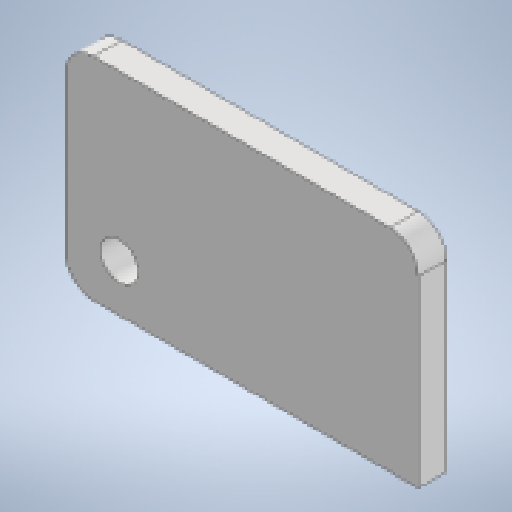
# Autodesk Inventor part: креп_центр_рейки
Saved by Autodesk Inventor 2023.1 (Build 271208000, 208)
## iProperties
Created: 2025-11-24
Part Number: креп_центр_рейки
Material: Типовые
Document SubType Name: Modeling
Designer: DELL
Density: 1 g/cm^3
Appearance: По умолчанию
Author: DELL
Autodesk Inventor part; units mm, degrees
ref_plane "YZ Plane" through (0, 0, 0) normal (1, 0, 0) x (0, 1, 0)
ref_plane "XZ Plane" through (0, 0, 0) normal (0, 1, 0) x (-1, 0, 0)
ref_plane "XY Plane" through (0, 0, 0) normal (0, 0, 1) x (1, 0, 0)
sketch "Эскиз1" plane through (0, 0, 0) normal (0, 0, 1) x (1, 0, 0)
  line L0 (112.2275, 7.2678) -> (167.2275, 7.2678)
  line L1 (167.2275, 7.2678) -> (167.2275, -32.7322)
  line L2 (167.2275, -32.7322) -> (112.2275, -32.7322)
  line L3 (112.2275, -32.7322) -> (112.2275, 7.2678)
  line L4 (112.2275, 7.2678) -> (167.2275, -32.7322) construction
  line L5 (167.2275, 7.2678) -> (112.2275, -32.7322) construction
  line L6 (147.2275, -32.7322) -> (167.2275, -32.7322)
  point P0 (139.7275, -12.7322)
  point P1 (139.7275, -32.7322)
  dimension "d55" = 40
  dimension "d67" = 55
  constraints: 14 end point, 3 midpoint, 2 parallel, 1 horizontal, 1 perpendicular, 1 point on line
  measures "d55" distance of L1.end L0.end
  measures "d67" distance of L0.start L0.end
extrude "Выдавливание1" add sketch "Эскиз1" along normal blind 4
sketch "Эскиз6" plane through (0, 0, 4) normal (0, 0, 1) x (1, 0, 0)
  line L0 (112.2275, -32.7322) -> (167.2275, -32.7322) construction
  line L1 (167.2275, 7.2678) -> (112.2275, 7.2678) construction
  line L2 (112.2275, 7.2678) -> (112.2275, -32.7322) construction
  circle A0 centre (120.2275, 0.5528) radius 2.65
  line L3 (167.2275, -32.7322) -> (167.2275, 7.2678) projected
  line L4 (112.2275, -32.7322) -> (167.2275, -32.7322) projected
  line L5 (139.7275, -32.7322) -> (139.7275, 7.2678) construction
  circle A1 centre (159.2275, 0.5528) radius 2.65
  line L6 (167.2275, 7.2678) -> (112.2275, 7.2678) projected
  line L7 (112.2275, 7.2678) -> (112.2275, -32.7322) projected
  circle A2 centre (120.2275, -25.7322) radius 2.65
  circle A3 centre (159.2275, -25.7322) radius 2.65
  point P0 (0, 0)
  dimension "d76" = 8
  dimension "d77" = 5.3
  dimension "d78" = 6.715
  dimension "d79" = 5.3
  dimension "d80" = 33
  constraints: 4 centre point, 2 end point, 2 midpoint, 2 symmetric about line, 1 other
  measures "d76" distance from line of L2 A0.centre
  measures "d77" diameter of A0
  measures "d78" distance from line of L1 A0.centre
  measures "d79" diameter of A2
  measures "d80" distance from line of L1 A2.centre
extrude "Выдавливание5" cut sketch "Эскиз6" against normal blind 4 contours A0 | A1 | A2 | A3
fillet "Сопряжение5" radius 4 4 edges at (112.2275, -32.7322, 2) (112.2275, 7.2678, 2) (167.2275, 7.2678, 2) (167.2275, -32.7322, 2)
